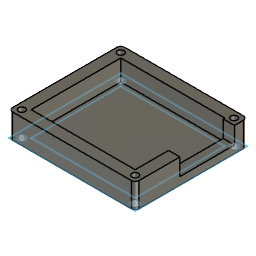
assembly (Autodesk Fusion 360 archive; units mm, degrees)
design "bottom"
part number: 2026-07-18-15-50-17-665
Autodesk Fusion 360 part; units mm, degrees
sketch "Sketch1" plane through (0, 0, 0) normal (0, 0, 1) x (1, 0, 0)
  line L0 (4.874, 50) -> (60, 50)
  line L1 (60, 50) -> (60, 2.5)
  line L2 (60, 2.5) -> (4.874, 2.5)
  line L3 (4.874, 2.5) -> (4.874, 50)
  line L4 (-1.126, 56) -> (66, 56)
  line L5 (66, 56) -> (66, -3.5)
  line L6 (66, -3.5) -> (-1.126, -3.5)
  line L7 (-1.126, -3.5) -> (-1.126, 56)
  circle A0 centre (2.374, 52.5) radius 1.75
  circle A1 centre (2.374, 0) radius 1.75
  circle A2 centre (62.5, 52.5) radius 1.75
  circle A3 centre (62.5, 0) radius 1.75
  dimension "d1" = 55.126
  dimension "d2" = 47.5
  dimension "d3" = 6
  dimension "d4" = 6
  dimension "d5" = 6
  dimension "d6" = 6
  dimension "d7" = 3.5
  dimension "d8" = 3.5
  dimension "d9" = 3.5
  dimension "d10" = 3.5
  dimension "d11" = 3.5
  dimension "d12" = 3.5
  dimension "d13" = 3.5
  dimension "d14" = 3.5
  dimension "d15" = 3.5
  dimension "d16" = 3.5
  dimension "d17" = 3.5
  dimension "d18" = 3.5
  constraint horizontal L0
  constraint vertical L1
  constraint horizontal L2
  constraint vertical L3
  constraint horizontal L4
  constraint vertical L5
  constraint horizontal L6
  constraint vertical L7
  measures "d1" distance of L1 L3
  measures "d2" distance of L0 L2
  measures "d3" distance of L0 L4
  measures "d4" distance of L3 L7
  measures "d5" distance of L1 L5
  measures "d6" distance of L2 L6
  measures "d7" diameter of A0
  measures "d8" distance of L4 A0.centre
  measures "d9" distance of L7 A0.centre
  measures "d10" diameter of A1
  measures "d11" distance of L6 A1.centre
  measures "d12" distance of L7 A1.centre
  measures "d13" diameter of A2
  measures "d14" distance of L4 A2.centre
  measures "d15" distance of L5 A2.centre
  measures "d16" diameter of A3
  measures "d17" distance of L5 A3.centre
  measures "d18" distance of L6 A3.centre
extrude "Extrude1" add sketch "Sketch1" along normal blind 13
extrude "Extrude2" add sketch "Sketch1" along normal blind 2 contours L0 L1 L2 L3
sketch "Sketch2" plane through (0, 0, 13) normal (0, 0, 1) x (-1, 0, 0)
  line L0 (-60, -2.5) -> (-4.874, -2.5)
  line L1 (-4.874, -2.5) -> (-4.874, -50)
  line L2 (-4.874, -50) -> (-60, -50)
  line L3 (-60, -50) -> (-60, -2.5)
  circle A0 centre (-62.5, -52.5) radius 1.75
  circle A1 centre (-2.374, -52.5) radius 1.75
  circle A2 centre (-2.374, 0) radius 1.75
  circle A3 centre (-62.5, 0) radius 1.75
  line L4 (1.126, 3.5) -> (-66, 3.5)
  line L5 (-66, 3.5) -> (-66, -56)
  line L6 (-66, -56) -> (1.126, -56)
  line L7 (1.126, -56) -> (1.126, 3.5)
  line L8 (-60, -49.1938) -> (-66, -49.1938)
  line L9 (-66, -49.1938) -> (-66, -20.1938)
  line L10 (-66, -20.1938) -> (-60, -20.1938)
  line L11 (-60, -20.1938) -> (-60, -49.1938)
  dimension "d23" = 29
  constraint horizontal L8
  constraint vertical L9
  constraint horizontal L10
  constraint vertical L11
  constraint coincident L5 L9.end
  constraint coincident L3 L8.start
  measures "d23" distance of L8 L10
extrude "Extrude3" cut sketch "Sketch2" against normal blind 9 contours L3 L5 L8 L9 L10 L11
fillet "Fillet1" radius 2 4 edges at (-1.126, 56, 6.5) (-1.126, -3.5, 6.5) (66, -3.5, 6.5) (66, 56, 6.5)

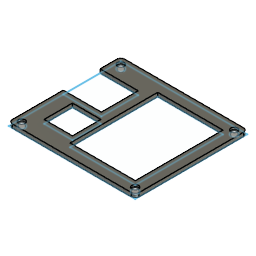
design "top"
part number: 2026-07-18-16-11-08-680
Autodesk Fusion 360 part; units mm, degrees
sketch "Sketch1" plane through (0, 0, 0) normal (0, 0, 1) x (1, 0, 0)
  line L0 (-17.126, 50.0374) -> (50, 50.0374)
  line L1 (50, 50.0374) -> (50, -9.4626)
  line L2 (50, -9.4626) -> (-17.126, -9.4626)
  line L3 (-17.126, -9.4626) -> (-17.126, 50.0374)
  circle A0 centre (-13.626, 46.5374) radius 1.75
  circle A1 centre (46.5, 46.5374) radius 1.75
  circle A2 centre (46.5, -5.9626) radius 1.75
  circle A3 centre (-13.626, -5.9626) radius 1.75
  line L4 (-17.1389, 39.0374) -> (3.0611, 39.0374)
  line L5 (3.0611, 39.0374) -> (3.0611, 19.5374)
  line L6 (3.0611, 19.5374) -> (-17.1389, 19.5374)
  line L7 (-17.1389, 19.5374) -> (-17.1389, 39.0374)
  line L8 (6.289, 16) -> (-8.711, 16)
  line L9 (-8.711, 16) -> (-8.711, 1)
  line L10 (-8.711, 1) -> (6.289, 1)
  line L11 (6.289, 1) -> (6.289, 16)
  line L12 (43.55, 43.4874) -> (8.95, 43.4874)
  line L13 (8.95, 43.4874) -> (8.95, -2.9126)
  line L14 (8.95, -2.9126) -> (43.55, -2.9126)
  line L15 (43.55, -2.9126) -> (43.55, 43.4874)
  dimension "d1" = 59.5
  dimension "d2" = 67.126
  dimension "d5" = 3.5
  dimension "d6" = 3.5
  dimension "d7" = 3.5
  dimension "d8" = 3.5
  dimension "d9" = 3.5
  dimension "d10" = 3.5
  dimension "d11" = 3.5
  dimension "d12" = 3.5
  dimension "d13" = 3.5
  dimension "d14" = 3.5
  dimension "d15" = 3.5
  dimension "d16" = 3.5
  dimension "d23" = 20.2
  dimension "d24" = 19.5
  dimension "d25" = 11
  dimension "d26" = 15
  dimension "d27" = 15
  dimension "d28" = 8.415
  dimension "d29" = 34.6
  dimension "d30" = 46.4
  dimension "d31" = 6.55
  dimension "d32" = 6.45
  constraint horizontal L0
  constraint vertical L1
  constraint horizontal L2
  constraint vertical L3
  constraint horizontal L4
  constraint vertical L5
  constraint horizontal L6
  constraint vertical L7
  constraint horizontal L8
  constraint vertical L9
  constraint horizontal L10
  constraint vertical L11
  constraint horizontal L12
  constraint vertical L13
  constraint horizontal L14
  constraint vertical L15
  measures "d1" distance of L0 L2
  measures "d2" distance of L1 L3
  measures "d5" diameter of A0
  measures "d6" distance of L0 A0.centre
  measures "d7" distance of L3 A0.centre
  measures "d8" diameter of A1
  measures "d9" distance of L1 A1.centre
  measures "d10" distance of L0 A1.centre
  measures "d11" diameter of A2
  measures "d12" distance of L1 A2.centre
  measures "d13" distance of L2 A2.centre
  measures "d14" diameter of A3
  measures "d15" distance of L2 A3.centre
  measures "d16" distance of L3 A3.centre
  measures "d23" distance of L5 L7
  measures "d24" distance of L4 L6
  measures "d25" distance of L0 L4
  measures "d26" distance of L8 L10
  measures "d27" distance of L9 L11
  measures "d28" distance of L3 L9.end
  measures "d29" distance of L13 L15
  measures "d30" distance of L12 L14
  measures "d31" distance of L0 L12.start
  measures "d32" distance of L1 L15
extrude "Extrude2" add sketch "Sketch1" along normal blind 2 contours L0 L1 L2 L3 L4 L5 L6
fillet "Fillet1" radius 2 4 edges at (50, -9.4626, 1) (-17.126, -9.4626, 1) (50, 50.0374, 1) (-17.126, 50.0374, 1)
extrude "Extrude3" add sketch "Sketch1" along normal blind 1 contours A0 | A1 | A2 | A3
